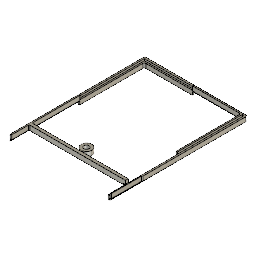
kradex z7 raiser 3mm 1.4 (Autodesk Fusion 360 design; units mm, degrees)
part number: 2025-09-26-18-23-52-872
Autodesk Fusion 360 part; units mm, degrees
sketch "Sketch1 base" plane through (0, 0, 0) normal (0, 0, 1) x (1, 0, 0)
  line L0 (34.225, 45.35) -> (-34.225, 45.35)
  line L1 (-34.225, 45.35) -> (-34.225, -45.35)
  line L2 (-34.225, -45.35) -> (34.225, -45.35)
  line L3 (34.225, -45.35) -> (34.225, 45.35)
  line L4 (34.225, 45.35) -> (-34.225, -45.35) construction
  line L5 (-34.225, 45.35) -> (34.225, -45.35) construction
  line L6 (34.225, 43) -> (-34.225, 43)
  line L7 (-32.075, 45.35) -> (-32.075, -45.35)
  line L8 (32.075, -45.35) -> (32.075, 45.35)
  line L9 (34.225, -0.15) -> (-34.225, -0.15)
  line L10 (34.225, -31.8) -> (-34.225, -31.8)
  line L11 (34.225, -33.8) -> (-34.225, -33.8)
  circle A0 centre (0, -0.15) radius 3.6
  circle A1 centre (0, -0.15) radius 1.75
  line L12 (34.225, -24.75) -> (-34.225, -24.75)
  line L13 (-33.7753, -24.75) -> (-33.7753, -45.35)
  line L14 (33.7759, -24.75) -> (33.7759, -45.35)
  dimension "d1" = 68.45
  dimension "d2" = 90.7
  dimension "d3" = -2.35
  dimension "d4" = -2.15
  dimension "d5" = -2.15
  dimension "d6" = -45.5
  dimension "d7" = -77.15
  dimension "d8" = -2
  dimension "d9" = 7.2
  dimension "d10" = 3.5
  dimension "d11" = 9.05
  constraint horizontal L0
  constraint perpendicular L0 L1
  constraint parallel L0 L2
  constraint parallel L1 L3
  constraint coincident L4 origin
  constraint coincident L5 origin
  constraint midpoint L9 A0.centre
  constraint concentric A0 A1
  constraint coincident L12 L13.start
  constraint perpendicular L12 L13
  constraint coincident L2 L13.end
  constraint coincident L12 L14.start
  constraint coincident L2 L14.end
  constraint perpendicular L2 L14
  measures "d1" distance of L1.end L2.end
  measures "d2" distance of L0.end L1.end
  measures "d9" diameter of A0
  measures "d10" diameter of A1
extrude "Extrude1" add sketch "Sketch1 base" along normal blind 3 contours L0 L3 L6 L8 | L0 L6 L7 L8 | L3 L6 L8 L9 | L0 L1 L6 L7 | L3 L8 L9 L12 | L1 L6 L7 L9 | L1 L7 L9 L12 | L8 L10 L12 L14 | L9 A0 A1 | L9 A0 A1 | L7 L10 L12 L13 | L8 L10 L11 L14 | L7 L8 L10 L11 | L7 L10 L11 L13 | L2 L8 L11 L14 | L2 L7 L11 L13 makes body 1 at (-10.6917, 44.5667, 0) makes body 2 at (3.5821, -0.5084, 1)
sketch "Sketch2 top" plane through (0, 0, 3) normal (0, 0, 1) x (-1, 0, 0)
  line L0 (-32.075, -43) -> (-32.075, 31.8)
  line L1 (-32.075, 31.8) -> (32.075, 31.8)
  line L2 (32.075, 31.8) -> (32.075, -43)
  line L3 (32.075, -43) -> (-32.075, -43)
  line L4 (-34.225, 24.75) -> (-34.225, -45.35)
  line L5 (-34.225, -45.35) -> (34.225, -45.35)
  line L6 (34.225, -45.35) -> (34.225, 24.75)
  line L7 (34.225, 24.75) -> (33.7753, 24.75)
  line L8 (33.7753, 24.75) -> (33.7753, 45.35)
  line L9 (33.7753, 45.35) -> (32.075, 45.35)
  line L10 (32.075, 45.35) -> (32.075, 33.8)
  line L11 (32.075, 33.8) -> (-32.075, 33.8)
  line L12 (-32.075, 33.8) -> (-32.075, 45.35)
  line L13 (-32.075, 45.35) -> (-33.7759, 45.35)
  line L14 (-33.7759, 45.35) -> (-33.7759, 24.75)
  line L15 (-33.7759, 24.75) -> (-34.225, 24.75)
  line L16 (34.225, 0.1491) -> (-34.225, 0.1491)
  line L17 (32.9252, 45.35) -> (32.075, 45.35)
  line L18 (32.075, 45.35) -> (32.075, -43.8588)
  line L19 (32.075, -43.8588) -> (32.9252, -43.8588)
  line L20 (0, -50) -> (0, -25)
  line L21 (32.075, -43) -> (-33.0751, -43)
  line L22 (-33.0751, -43) -> (-33.0751, -44)
  line L23 (-33.0751, -44) -> (32.075, -44)
  line L24 (32.075, -44) -> (32.075, -43)
  line L25 (-32.075, 45.35) -> (-33, 45.35)
  line L26 (-33.0751, -43) -> (-32.075, -43)
  line L27 (-32.075, -43) -> (-32.075, 45.35)
  line L28 (32.075, -44) -> (33.075, -44)
  line L29 (33.075, -44) -> (33.075, 45.35)
  line L30 (33.075, 45.35) -> (32.075, 45.35)
  line L31 (32.075, 45.35) -> (32.075, -44)
  line L32 (-32.075, -43) -> (-33.075, -43)
  line L33 (-33.075, -43) -> (-33.075, 45.35)
  line L34 (-33.075, 45.35) -> (-32.075, 45.35)
  line L35 (-32.075, 45.35) -> (-32.075, -43)
  dimension "d14" = 1
  dimension "d15" = 1
  constraint coincident L6 L16.start
  constraint coincident L4 L16.end
  constraint perpendicular L4 L16
  constraint horizontal L17
  constraint vertical L18
  constraint horizontal L19
  constraint midpoint L9 L17.start
  constraint perpendicular L3 L20
  constraint horizontal L21
  constraint vertical L22
  constraint horizontal L23
  constraint vertical L24
  constraint coincident L2.end L3.start
  constraint horizontal L25
  constraint horizontal L26
  constraint vertical L27
  constraint coincident L12.end L13.start
  constraint horizontal L28
  constraint vertical L29
  constraint horizontal L30
  constraint vertical L31
  constraint coincident L9 L29.end
  constraint horizontal L32
  constraint vertical L33
  constraint horizontal L34
  constraint vertical L35
  constraint coincident L25 L33.end
  measures "d14" distance of L23.end L28.end
  measures "d15" distance of L0.start L32.end
extrude "Extrude2" add sketch "Sketch2 top" along normal blind 1.25 contours L0 L16 L21 L26 L27 L32 L33 L35 | L3 L20 L21 L22 L23 L26 L32 bodies 1
extrude "Extrude3" add sketch "Sketch2 top" along normal blind 1.25 contours L2 L9 L10 L16 L17 L18 L29 L30 L31 bodies 1
extrude "Extrude4" cut sketch "Sketch2 top" against normal blind 1.25 contours L3 L18 L20 L21 L23 L24 L31 | L2 L16 L18 L24 L28 L29 L31 bodies 1
extrude "Extrude5" cut sketch "Sketch2 top" against normal blind 1.25 contours L0 L12 L13 L16 L25 L27 L33 L34 L35 bodies 1
extrude "Extrude6" add sketch "Sketch2 top" along normal blind 1.25 contours L1 L11 L18 L27 L31 L35 bodies 1
sketch "Sketch3 bottom" plane through (0, 0, 0) normal (0, 0, -1) x (1, 0, 0)
  line L0 (32.075, 31.8) -> (32.075, -43)
  line L1 (32.075, -43) -> (-32.075, -43)
  line L2 (-32.075, -43) -> (-32.075, 31.8)
  line L3 (-32.075, 31.8) -> (32.075, 31.8)
  line L4 (34.225, -45.35) -> (34.225, 24.75)
  line L5 (34.225, 24.75) -> (33.7759, 24.75)
  line L6 (33.7759, 24.75) -> (33.7759, 45.35)
  line L7 (33.7759, 45.35) -> (32.075, 45.35)
  line L8 (32.075, 45.35) -> (32.075, 33.8)
  line L9 (32.075, 33.8) -> (-32.075, 33.8)
  line L10 (-32.075, 33.8) -> (-32.075, 45.35)
  line L11 (-32.075, 45.35) -> (-33.7753, 45.35)
  line L12 (-33.7753, 45.35) -> (-33.7753, 24.75)
  line L13 (-33.7753, 24.75) -> (-34.225, 24.75)
  line L14 (-34.225, 24.75) -> (-34.225, -45.35)
  line L15 (-34.225, -45.35) -> (34.225, -45.35)
  line L16 (34.225, 0.1493) -> (-34.225, 0.1493)
  line L17 (0, -49) -> (0, -39)
  line L18 (32.075, -43) -> (33.075, -43)
  line L19 (33.075, -43) -> (33.075, 45.35)
  line L20 (33.075, 45.35) -> (32.075, 45.35)
  line L21 (32.075, 45.35) -> (32.075, -43)
  line L22 (-32.075, -43) -> (-33.075, -43)
  line L23 (-33.075, -43) -> (-33.075, 45.35)
  line L24 (-33.075, 45.35) -> (-32.075, 45.35)
  line L25 (-32.075, 45.35) -> (-32.075, -43)
  line L26 (-33.075, -43) -> (33.0749, -43)
  line L27 (33.0749, -43) -> (33.0749, -44)
  line L28 (33.0749, -44) -> (-33.075, -44)
  line L29 (-33.075, -44) -> (-33.075, -43)
  dimension "d26" = 1
  dimension "d27" = 1
  dimension "d28" = 1
  constraint coincident L4 L16.start
  constraint coincident L14 L16.end
  constraint perpendicular L1 L17
  constraint horizontal L18
  constraint vertical L19
  constraint horizontal L20
  constraint vertical L21
  constraint coincident L7 L19.end
  constraint coincident L0.end L1.start
  constraint horizontal L22
  constraint vertical L23
  constraint horizontal L24
  constraint vertical L25
  constraint coincident L11 L23.end
  constraint coincident L1.end L2.start
  constraint horizontal L26
  constraint vertical L27
  constraint horizontal L28
  constraint vertical L29
  measures "d26" distance of L0.end L18.end
  measures "d27" distance of L1.end L22.end
  measures "d28" distance of L22.end L28.end
extrude "Extrude7" add sketch "Sketch3 bottom" along normal blind 1.25 contours L2 L16 L22 L23 L25 L26 | L1 L17 L22 L26 L28 L29 bodies 1
extrude "Extrude8" cut sketch "Sketch3 bottom" against normal blind 1.25 contours L0 L16 L18 L19 L21 L26 | L1 L17 L18 L26 L27 L28 bodies 1
extrude "Extrude9" cut sketch "Sketch3 bottom" against normal blind 1.25 contours L2 L10 L11 L16 L23 L24 L25 bodies 1
extrude "Extrude10" add sketch "Sketch3 bottom" along normal blind 1.25 contours L0 L7 L8 L16 L19 L20 L21 bodies 1
extrude "Extrude11" cut sketch "Sketch3 bottom" against normal blind 1 contours L3 L9 L21 L25 bodies 1
fillet "Fillet1" radius 1 1 edges at (34.225, 45.35, 1.5) on bodies 1
fillet "Fillet2" radius 0.5 2 edges at (33.7759, -45.35, 1.5) (-33.7753, -45.35, 1.5) on bodies 1
fillet "Fillet3" radius 1 1 edges at (-34.225, 45.35, 1.5) on bodies 1
fillet "Fillet4" radius 1 1 edges at (32.075, 43, 2.75) on bodies 1
fillet "Fillet5" radius 1 1 edges at (-32.075, 43, 0.25) on bodies 1
fillet "Fillet6" radius 0.5 2 edges at (-32.075, -33.8, 2.75) (-32.075, -31.8, 2.75) on bodies 1
fillet "Fillet7" radius 1.5 1 edges at (32.075, -33.8, 1.375) on bodies 1
fillet "Fillet8" radius 1.5 1 edges at (32.075, -31.8, 1.375) on bodies 1
fillet "Fillet9" radius 0.5 1 edges at (34.225, -24.75, 1.5) on bodies 1
fillet "Fillet10" radius 0.5 1 edges at (-34.225, -24.75, 1.5) on bodies 1
fillet "Fillet11" radius 0.5 1 edges at (-33.075, 44, -0.625) on bodies 1
fillet "Fillet12" radius 0.5 1 edges at (33.0751, 44, 3.625) on bodies 1
move_body "Move1" bodies 2 to x (1, 0, 0) y (0, 1, 0) z (0, 0, 1) at (0, 0, 1.25)
sketch "Sketch4" plane through (0, 0, 0) normal (0, 0, 1) x (1, 0, 0)
  line L0 (-0.5, -31.8) -> (0.5, -31.8)
  line L1 (0.5, -31.8) -> (0.5, -30.8)
  line L2 (0.5, -30.8) -> (-0.5, -30.8)
  line L3 (-0.5, -30.8) -> (-0.5, -31.8)
  dimension "d63" = 1
  dimension "d64" = 1
  constraint horizontal L0
  constraint vertical L1
  constraint horizontal L2
  constraint vertical L3
  measures "d63" distance of L0.start L0.end
  measures "d64" distance of L0.start L2.end
extrude "Extrude12" add sketch "Sketch4" along normal blind 4.25 bodies 1
extrude "Extrude13" cut 1 faces at (-0.1667, -31.1333, 0) along direction (0, 0, 1) blind 3 on bodies 1 bodies 1
move_body "Move2" bodies 2 to x (1, 0, 0) y (0, 1, 0) z (0, 0, 1) at (0, -27.5, 0)
move_face "MoveFace1" by (-1, 0, 0) 1 faces at (2.9634, -27.3842, 4.25) on bodies 2
combine "Combine1" operation add target body 1 tool bodies 2
